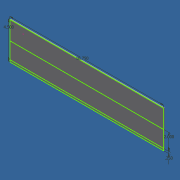
# Autodesk Inventor part: circuit board
Saved by Autodesk Inventor 2012 (Build 160160000, 160)
## iProperties
Created: 2012-02-03
Part Number: circuit board
Material: Default
Document SubType Name: Modeling
Designer: Allison Garza
Density: 1 g/cm^3
Author: Allison Garza
Autodesk Inventor part; units mm, degrees
ref_plane "YZ Plane" through (0, 0, 0) normal (1, 0, 0) x (0, 1, 0)
ref_plane "XZ Plane" through (0, 0, 0) normal (0, 1, 0) x (-1, 0, 0)
ref_plane "XY Plane" through (0, 0, 0) normal (0, 0, 1) x (1, 0, 0)
sketch "Sketch1" plane through (0, 0, 0) normal (0, 0, 1) x (1, 0, 0)
  line L0 (-41.6667, 18.4708) -> (434.5833, 18.4708)
  line L1 (434.5833, 18.4708) -> (434.5833, -95.8292)
  line L2 (434.5833, -95.8292) -> (-41.6667, -95.8292)
  line L3 (-41.6667, -95.8292) -> (-41.6667, 18.4708)
  line L4 (-41.6667, -38.6792) -> (434.5833, -38.6792)
  line L5 (-41.6667, -89.4792) -> (434.5833, -89.4792)
  point P0 (0, 0)
  dimension "d0" = 476.25
  dimension "d1" = 114.3
  dimension "d5" = 6.35
  dimension "d6" = 50.8
  constraints: 12 end point, 3 perpendicular, 2 midpoint, 2 parallel, 2 point on line, 1 horizontal
  measures "d0" distance of L0.start L0.end
  measures "d1" distance of L2.end L0.start
  measures "d5" distance of L1.end L5.end
  measures "d6" distance of L5.end L4.end
extrude "Extrusion1" add sketch "Sketch1" against normal blind 3.175
body "Solid1"
